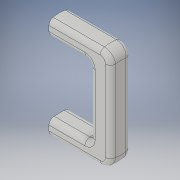
# Autodesk Inventor part: wheel grip
Saved by Autodesk Inventor 2018 (Build 220112000, 112)
## iProperties
Created: 2018-08-08
Part Number: wheel grip
Material: Generic
Document SubType Name: Modeling
Designer: Cole Tucker
Density: 1 g/cm^3
Appearance: Default
Author: Cole Tucker
Autodesk Inventor part; units mm, degrees
ref_plane "YZ Plane" through (0, 0, 0) normal (1, 0, 0) x (0, 1, 0)
ref_plane "XZ Plane" through (0, 0, 0) normal (0, 1, 0) x (-1, 0, 0)
ref_plane "XY Plane" through (0, 0, 0) normal (0, 0, 1) x (1, 0, 0)
sketch "Sketch1" plane through (0, 0, 0) normal (1, 0, 0) x (0, 1, 0)
  line L0 (0, 0) -> (63.5, 0) construction
  line L1 (0, 0) -> (25.4, 0) construction
  line L2 (0, 0) -> (0, -12.7) construction
  line L3 (0, 0) -> (0, 12.7) construction
  line L4 (0, 12.7) -> (61.321, 12.7)
  line L5 (0, -12.7) -> (61.321, -12.7)
  arc A0 (61.321, -12.7) -> (61.321, 12.7) centre (25.4, 0) ccw
  line L6 (0, 12.7) -> (-61.321, 12.7)
  line L7 (0, -12.7) -> (-61.321, -12.7)
  arc A1 (-61.321, 12.7) -> (-61.321, -12.7) centre (-25.4, 0) ccw
  dimension "d0" = 63.5
  dimension "d1" = 25.4
  dimension "d2" = 12.7
  dimension "d3" = 12.7
  constraints: 16 end point, 5 point on circle, 3 horizontal, 3 symmetric about line, 2 centre point, 1 coincident, 1 perpendicular, 1 point on line, 1 vertical, 1 other
  measures "d0" distance of L0.start L0.end
  measures "d1" distance of L0.start L1.end
  measures "d2" distance of L0.start L2.end
  measures "d3" distance of L0.start L3.end
extrude "Extrusion1" add sketch "Sketch1" along normal blind 76.2
fillet "Fillet1" radius 12.7 2 edges at (76.2, 63.5, 0) (76.2, -63.5, 0)
fillet "Fillet2" radius 6.35 12 edges at (72.7389, 57.0619, 12.7) (76.2, -23.6985, 12.7) (76.2, 23.6985, 12.7) (72.7389, -57.0619, 12.7) (31.75, -61.321, 12.7) (31.75, 61.321, 12.7) (72.7389, 57.0619, -12.7) (76.2, -23.6985, -12.7) (76.2, 23.6985, -12.7) (72.7389, -57.0619, -12.7) (31.75, -61.321, -12.7) (31.75, 61.321, -12.7)
sketch "Sketch2" plane through (0, -56.5085, 12.7) normal (0, 0, 1) x (1, 0, 0)
  line L0 (0, -6.2217) -> (0, 0) construction
  line L1 (0, -6.2217) -> (0, 12.8283) construction
  line L2 (0, 113.017) -> (0, 0) construction
  line L3 (0, 113.017) -> (0, 119.2387) construction
  line L4 (0, 119.2387) -> (0, 100.1887) construction
  line L5 (0, 100.1887) -> (50.8, 100.1887)
  line L6 (50.8, 100.1887) -> (50.8, 12.5587)
  line L7 (50.8, 12.5587) -> (0, 12.5587)
  line L8 (0, 12.5587) -> (0, 100.1887)
  point P0 (0, 56.5085)
  dimension "d10" = 19.05
  dimension "d11" = 19.05
  dimension "d12" = 50.8
  dimension "d17" = 87.63
  constraints: 12 end point, 2 parallel, 2 point on line, 1 horizontal, 1 perpendicular
  measures "d10" distance of L0.start L1.end
  measures "d11" distance of L3.end L4.end
  measures "d12" distance of L6.end L7.end
  measures "d17" distance of L5.end L6.end
extrude "Extrusion2" cut sketch "Sketch2" against normal blind 76.2
fillet "Fillet3" radius 6.35 2 edges at (50.8, 43.6802, 0) (50.8, -43.9498, 0)
fillet "Fillet4" radius 6.35 10 edges at (48.9401, 41.8204, 12.7) (50.8, -0.1348, 12.7) (48.9401, -42.0899, 12.7) (22.225, -43.9498, 12.7) (22.225, 43.6802, 12.7) (48.9401, 41.8204, -12.7) (50.8, -0.1348, -12.7) (48.9401, -42.0899, -12.7) (22.225, -43.9498, -12.7) (22.225, 43.6802, -12.7)
body "Solid1"
